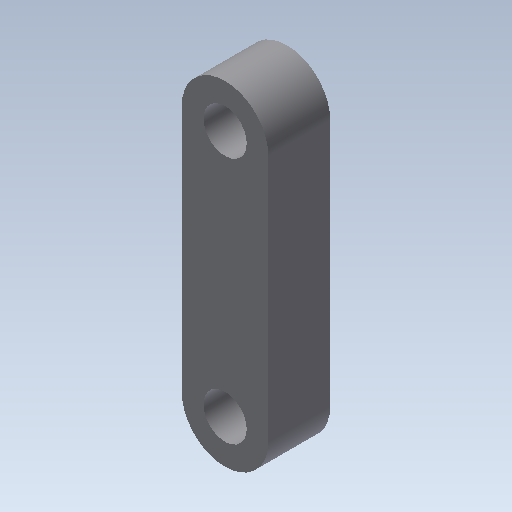
# Autodesk Inventor part: barMini
Saved by Autodesk Inventor 2020.1 (Build 241239000, 239)
## iProperties
Created: 2016-10-14
Part Number: barMini
Material: Generic
Document SubType Name: Modeling
Designer: Bardo91
Density: 1 g/cm^3
Appearance: Default
Author: Bardo91
Autodesk Inventor part; units mm, degrees
ref_plane "YZ Plane" through (0, 0, 0) normal (1, 0, 0) x (0, 1, 0)
ref_plane "XZ Plane" through (0, 0, 0) normal (0, 1, 0) x (-1, 0, 0)
ref_plane "XY Plane" through (0, 0, 0) normal (0, 0, 1) x (1, 0, 0)
sketch "Sketch1" plane through (0, 0, 0) normal (0, 0, 1) x (1, 0, 0)
  circle A0 centre (0, 0) radius 3.5
  line L0 (0, 0) -> (0, 20)
  circle A1 centre (0, 20) radius 3.5
  line L1 (-3.5, 20) -> (-3.5, 0)
  line L2 (0, 20) -> (3.5, 20)
  line L3 (3.5, 20) -> (3.5, 0)
  dimension "d0" = 7
  dimension "d1" = 20
  dimension "d2" = 7
  constraints: 8 end point, 5 point on circle, 2 centre point, 2 coincident, 2 tangent, 1 horizontal, 1 perpendicular, 1 vertical
  measures "d0" diameter of A0
  measures "d1" distance of L0.start L0.end
  measures "d2" diameter of A1
extrude "Extrusion1" add sketch "Sketch1" along normal blind 5
sketch "Sketch2" plane through (0, 0, 5) normal (0, 0, 1) x (1, 0, 0)
  arc A0 (3.5, 20) -> (-3.5, 20) centre (0, 20) ccw projected
  circle A1 centre (0, 20) radius 1.75
  arc A2 (-3.5, 0) -> (3.5, 0) centre (0, 0) ccw projected
  circle A3 centre (0, 0) radius 1.75
  dimension "d5" = 3.5
  dimension "d6" = 3.5
  constraints: 2 centre point, 2 coincident
  measures "d5" diameter of A1
  measures "d6" diameter of A3
extrude "Extrusion2" cut sketch "Sketch2" against normal blind 5
body "Solid1"
